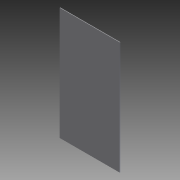
# Autodesk Inventor part: Door
Saved by Autodesk Inventor 2012 (Build 160160000, 160)
## iProperties
Created: 2012-04-20
Part Number: Door
Material: Default
Document SubType Name: Modeling
Designer: Puzzles
Density: 1 g/cm^3
Author: Puzzles
Autodesk Inventor part; units mm, degrees
ref_plane "YZ Plane" through (0, 0, 0) normal (1, 0, 0) x (0, 1, 0)
ref_plane "XZ Plane" through (0, 0, 0) normal (0, 1, 0) x (-1, 0, 0)
ref_plane "XY Plane" through (0, 0, 0) normal (0, 0, 1) x (1, 0, 0)
sketch "Sketch1" plane through (0, 0, 0) normal (0, 0, 1) x (1, 0, 0)
  line L0 (-152.4, 285.75) -> (152.4, 285.75)
  line L1 (152.4, 285.75) -> (152.4, -285.75)
  line L2 (152.4, -285.75) -> (-152.4, -285.75)
  line L3 (-152.4, -285.75) -> (-152.4, 285.75)
  point P0 (0, 0)
  point P1 (152.4, 0)
  point P2 (0, 285.75)
  dimension "d0" = 304.8
  dimension "d1" = 571.5
  constraints: 8 end point, 2 midpoint, 2 parallel, 1 horizontal, 1 horizontal alignment, 1 perpendicular, 1 vertical alignment
  measures "d0" distance of L0.start L0.end
  measures "d1" distance of L2.end L0.start
extrude "Extrusion1" add sketch "Sketch1" along normal blind 3
body "Solid1"
